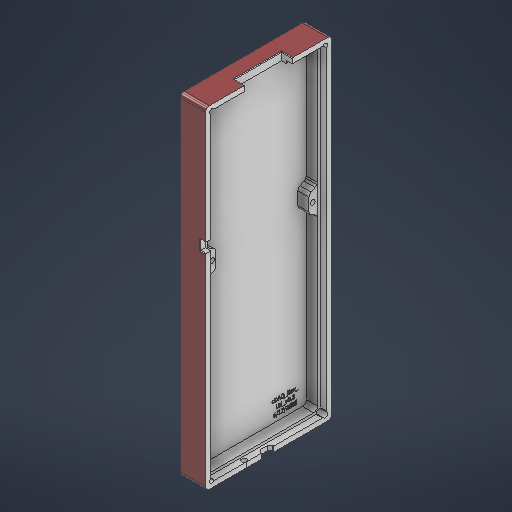
# Autodesk Inventor part: cDAQ_Box_Lid_v0.2
Saved by Autodesk Inventor 2027 (Build 310192000, 192)
## iProperties
Created: 2026-05-08
Part Number: cDAQ_Box_Lid_v0.2
Material: Generic
Document SubType Name: Modeling
Designer: giese
Density: 1 g/cm^3
Appearance: Default
Author: giese
Autodesk Inventor part; units mm, degrees
(part 1 of 2)
ref_plane "YZ Plane" through (0, 0, 0) normal (1, 0, 0) x (0, 1, 0)
ref_plane "XZ Plane" through (0, 0, 0) normal (0, 1, 0) x (-1, 0, 0)
ref_plane "XY Plane" through (0, 0, 0) normal (0, 0, 1) x (1, 0, 0)
sketch "Sketch1" plane through (0, 0, 0) normal (1, 0, 0) x (0, 1, 0)
  line L0 (50.7569, 48.4212) -> (-216.9591, 48.4212)
  line L1 (-216.9591, 48.4212) -> (-216.9591, -53.1788)
  line L2 (-216.9591, -53.1788) -> (50.7569, -53.1788)
  line L3 (50.7569, -53.1788) -> (50.7569, 48.4212)
  point P0 (0, 0)
  dimension "d0" = 101.6
  dimension "d1" = 267.716
  constraints: 8 end point, 2 parallel, 1 horizontal, 1 perpendicular
  measures "d0" distance of L2.end L0.start
  measures "d1" distance of L0.start L0.end
extrude "Extrusion1" add sketch "Sketch1" along normal blind 20.32
sketch "Sketch2" plane through (20.32, 0, 0) normal (1, 0, 0) x (0, 0, -1)
  line L0 (-42.0712, 44.4069) -> (46.8288, 44.4069)
  line L1 (46.8288, 44.4069) -> (46.8288, -210.6091)
  line L2 (46.8288, -210.6091) -> (-42.0712, -210.6091)
  line L3 (-42.0712, -210.6091) -> (-42.0712, 44.4069)
  line L4 (-48.4212, 50.7569) -> (-48.4212, -216.9591) projected
  line L5 (-48.4212, -216.9591) -> (53.1788, -216.9591) projected
  point P0 (0, 0)
  dimension "d4" = 88.9
  dimension "d5" = 255.016
  dimension "d6" = 6.35
  dimension "d7" = 6.35
  constraints: 8 end point, 2 parallel, 1 horizontal, 1 perpendicular
  measures "d4" distance of L0.start L0.end
  measures "d5" distance of L0.end L1.end
  measures "d6" distance between parallel lines of L4 L3
  measures "d7" distance between parallel lines of L5 L2
extrude "Extrusion2" cut sketch "Sketch2" against normal blind 13.97
sketch "Sketch3" plane through (0, 0, 0) normal (-1, 0, 0) x (0, 0, 1)
  circle A0 centre (-30.3188, 7.3229) radius 2
  line L0 (-53.1788, -216.9591) -> (-53.1788, 50.7569) projected
  line L1 (-53.1788, 50.7569) -> (48.4212, 50.7569) projected
  circle A1 centre (-11.82, 7.3229) radius 2
  circle A2 centre (6.6789, 7.3229) radius 2
  point P0 (0, 0)
  dimension "d10" = 22.86
  dimension "d11" = 43.434
  dimension "d12" = 43.434
  dimension "d13" = 18.4988
  dimension "d14" = 4
  dimension "d15" = 4
  dimension "d16" = 43.434
  dimension "d17" = 18.4988
  dimension "d18" = 36.9976
  dimension "d21" = 4
  constraints: 3 centre point
  measures "d10" distance from line of L0 A0.centre
  measures "d11" distance from line of L1 A0.centre
  measures "d12" distance from line of L1 A1.centre
  measures "d13" distance of A0.centre A1.centre
  measures "d14" diameter of A1
  measures "d15" diameter of A2
  measures "d16" distance from line of L1 A2.centre
  measures "d17" distance of A1.centre A2.centre
  measures "d18" distance of A0.centre A2.centre
  measures "d21" diameter of A0
extrude "Extrusion3" [suppressed]
sketch "Sketch6" plane through (0, 50.7569, 48.4212) normal (0, 1, 0) x (1, 0, 0)
  line L0 (20.32, 6.35) -> (20.32, 95.25) projected
  line L1 (11.684, 31.75) -> (20.32, 31.75)
  line L2 (20.32, 31.75) -> (20.32, 69.85)
  line L3 (20.32, 69.85) -> (11.684, 69.85)
  line L4 (11.684, 69.85) -> (11.684, 31.75)
  line L5 (0, 101.6) -> (20.32, 101.6) projected
  point P0 (0, 48.4212)
  point P1 (16.002, 69.85)
  point P2 (16.002, 31.75)
  dimension "d30" = 8.636
  dimension "d31" = 38.1
  dimension "d32" = 31.75
  constraints: 8 end point, 2 midpoint, 2 parallel, 1 horizontal, 1 perpendicular, 1 point on line
  measures "d30" distance between parallel lines of L0 L4
  measures "d31" distance of point (16.002, 69.85) point (16.002, 31.75)
  measures "d32" distance between parallel lines of L5 L3
extrude "Extrusion5" cut sketch "Sketch6" against normal blind 6.35
fillet "Fillet1" radius 3.175 4 edges at (10.16, 50.7569, -53.1788) (10.16, 50.7569, 48.4212) (10.16, -216.9591, 48.4212) (10.16, -216.9591, -53.1788)
sketch "Sketch7" plane through (20.32, 0, 0) normal (1, 0, 0) x (0, 0, -1)
  line L0 (-42.0712, -210.6091) -> (-42.0712, 44.4069) projected
  line L1 (-42.0712, 44.4069) -> (-42.3252, 44.4069)
  line L2 (-42.3252, 46.5659) -> (-44.2302, 46.5659)
  line L3 (-44.2302, 46.5659) -> (-44.2302, 51.0109)
  line L4 (-42.0712, -190.1621) -> (-42.0712, -210.6091)
  line L5 (46.8288, -210.6091) -> (-42.0712, -210.6091) projected
  line L6 (-40.4202, -212.7681) -> (-44.2302, -212.7681)
  line L7 (-44.2302, -212.7681) -> (-44.2302, -190.1621)
  line L8 (46.8288, 44.4069) -> (46.8288, -210.6091) projected
  line L9 (46.8288, -192.7021) -> (46.8288, -210.6091)
  line L10 (46.8288, -210.6091) -> (43.9078, -210.6091)
  line L11 (46.8288, -210.6091) -> (46.8288, -192.7021)
  line L12 (48.9878, -192.7021) -> (48.9878, -212.7681)
  line L13 (48.9878, -212.7681) -> (43.9078, -212.7681)
  line L14 (-42.0712, 44.4069) -> (46.8288, 44.4069) projected
  line L15 (42.0028, 44.4069) -> (46.8288, 44.4069)
  line L16 (48.9878, 48.4709) -> (48.9878, 46.5659)
  line L17 (48.9878, 46.5659) -> (42.0028, 46.5659)
  line L18 (-42.3252, 46.5659) -> (42.0028, 46.5659)
  line L19 (42.0028, 44.4069) -> (-42.3252, 44.4069)
  line L20 (48.9878, 48.4709) -> (48.9878, -192.7021)
  line L21 (44.2888, -195.2421) -> (44.2888, 44.4069)
  line L22 (43.9078, -210.6091) -> (-40.4202, -210.6091)
  line L23 (-40.4202, -212.7681) -> (43.9078, -212.7681)
  line L24 (-44.2302, -190.1621) -> (-44.2302, 51.0109)
  line L25 (-42.0712, 44.4069) -> (-42.0712, -190.1621)
  point P0 (0, 0)
  point P1 (-42.0712, 51.0109)
  point P2 (-44.2302, 48.9789)
  point P3 (46.8288, 48.4709)
  point P4 (48.9878, 46.5659)
  point P5 (-44.2302, 46.5659)
  dimension "d34" = 2.159
  dimension "d35" = 2.159
  dimension "d38" = 2.159
  dimension "d39" = 2.159
  dimension "d42" = 2.159
  dimension "d43" = 2.159
  dimension "d46" = 2.159
  dimension "d47" = 2.159
  constraints: 44 end point, 9 point on line, 4 parallel, 4 perpendicular, 2 collinear, 2 horizontal, 2 vertical
  measures "d34" distance between parallel lines of L2 L1
  measures "d35" distance between parallel lines of L0 L3
  measures "d38" distance between parallel lines of L7 L0
  measures "d39" distance between parallel lines of L5 L6
  measures "d42" distance between parallel lines of L5 L13
  measures "d43" distance between parallel lines of L8 L12
  measures "d46" distance between parallel lines of L14 L17
  measures "d47" distance between parallel lines of L8 L16
extrude "Extrusion6" cut sketch "Sketch7" against normal blind 5 contours L0 L14 L8 L5 | L18 L17 L20 L12 L13 L23 L6 L7 L24 L2
fillet "Fillet2" radius 3.175 6 edges at (10.835, 44.4069, 42.0712) (10.835, 44.4069, -46.8288) (10.835, -210.6091, 42.0712) (17.82, -212.7681, 44.2302) (10.835, -210.6091, -46.8288) (17.82, -212.7681, -48.9878)
sketch "Sketch11" plane through (15.32, 0, 0) normal (1, 0, 0) x (0, 0, -1)
  circle A0 centre (48.0988, 45.6769) radius 1.9939
  line L0 (50.0038, 50.7569) -> (21.4288, 50.7569) projected
  line L1 (53.1788, -213.7841) -> (53.1788, 47.5819) projected
  arc A1 (46.9238, 45.7719) -> (43.7488, 48.9469) centre (43.7488, 45.7719) ccw projected
  circle A2 centre (-43.3412, 45.6769) radius 1.9939
  line L2 (-48.4212, 47.5819) -> (-48.4212, -213.7841) projected
  line L3 (-16.6712, 50.7569) -> (-45.2462, 50.7569) projected
  circle A3 centre (48.0988, -211.8791) radius 1.9939
  line L4 (-45.2462, -216.9591) -> (50.0038, -216.9591) projected
  circle A4 centre (-43.3412, -211.8791) radius 1.9939
  circle A5 centre (43.0188, -63.5431) radius 1.9939
  circle A6 centre (-38.2612, -63.5431) radius 1.9939
  point P0 (0, 0)
  point P1 (45.9939, 48.017)
  point P2 (48.5528, -43.2993)
  point P3 (45.3778, -46.4743)
  point P4 (-30.4007, -42.8803)
  point P5 (-33.5757, -46.0553)
  dimension "d58" = 3.9878
  dimension "d59" = 5.08
  dimension "d60" = 5.08
  dimension "d61" = 3.9878
  dimension "d62" = 3.9878
  dimension "d63" = 5.08
  dimension "d64" = 5.08
  dimension "d65" = 3.9878
  dimension "d66" = 5.08
  dimension "d67" = 5.08
  dimension "d76" = 5.08
  dimension "d77" = 5.08
  dimension "d114" = 3.9878
  dimension "d115" = 114.3
  dimension "d116" = 10.16
  dimension "d117" = 3.9878
  dimension "d118" = 114.3
  dimension "d119" = 10.16
  constraints: 6 centre point, 1 point on circle
  measures "d58" diameter of A0
  measures "d59" distance from line of L2 A2.centre
  measures "d60" distance from line of L3 A2.centre
  measures "d61" diameter of A2
  measures "d62" diameter of A3
  measures "d63" distance from line of L1 A3.centre
  measures "d64" distance from line of L4 A3.centre
  measures "d65" diameter of A4
  measures "d66" distance from line of L2 A4.centre
  measures "d67" distance from line of L4 A4.centre
  measures "d76" distance from line of L1 A0.centre
  measures "d77" distance from line of L0 A0.centre
  measures "d114" diameter of A5
  measures "d115" distance from line of A5.centre L0
  measures "d116" distance from line of L1 A5.centre
  measures "d117" diameter of A6
  measures "d118" distance from line of A6.centre L3
  measures "d119" distance from line of L2 A6.centre
extrude "Extrusion8" cut sketch "Sketch11" along normal blind 5.08 and the other way blind 17.78
sketch "Sketch13" plane through (6.35, 0, 0) normal (1, 0, 0) x (0, 0, -1)
  line L0 (17.2683, -193.8209) -> (42.3242, -193.8209) construction
  line L1 (42.3242, -193.8209) -> (42.3242, -202.6852) construction
  line L2 (42.3242, -202.6852) -> (17.2683, -202.6852) construction
  line L3 (17.2683, -202.6852) -> (17.2683, -193.8209) construction
  spline S0 degree 2 poles (20.1261, -196.985) (19.889, -196.985) (19.4963, -196.8393) (19.3555, -196.6911) knots 0 0 0 1 2 2 2
  spline S1 degree 2 poles (19.3555, -196.6911) (19.2147, -196.5454) (19.0591, -196.0958) (19.0591, -195.7945) knots 0 0 0 1 2 2 2
  spline S2 degree 2 poles (19.0591, -195.7945) (19.0591, -195.4931) (19.2196, -195.0535) (19.3555, -194.9053) knots 0 0 0 1 2 2 2
  spline S3 degree 2 poles (19.3555, -194.9053) (19.4913, -194.7546) (19.8939, -194.5941) (20.1261, -194.5941) knots 0 0 0 1 2 2 2
  spline S4 degree 2 poles (20.1261, -194.5941) (20.3138, -194.5941) (20.6646, -194.7003) (20.8004, -194.7694) knots 0 0 0 1 2 2 2
  line L4 (20.8004, -194.7694) -> (20.8004, -195.2017)
  line L5 (20.8004, -195.2017) -> (20.7782, -195.2017)
  spline S5 degree 2 poles (20.7782, -195.2017) (20.7362, -195.1671) (20.6078, -195.0782) (20.5164, -195.0312) knots 0 0 0 1 2 2 2
  spline S6 degree 2 poles (20.5164, -195.0312) (20.4349, -194.9917) (20.2175, -194.93) (20.1187, -194.93) knots 0 0 0 1 2 2 2
  spline S7 degree 2 poles (20.1187, -194.93) (19.8198, -194.93) (19.4568, -195.382) (19.4568, -195.7945) knots 0 0 0 1 2 2 2
  spline S8 degree 2 poles (19.4568, -195.7945) (19.4568, -196.1971) (19.8075, -196.6491) (20.1187, -196.6491) knots 0 0 0 1 2 2 2
  spline S9 degree 2 poles (20.1187, -196.6491) (20.3064, -196.6491) (20.6473, -196.4935) (20.7782, -196.3725) knots 0 0 0 1 2 2 2
  line L6 (20.7782, -196.3725) -> (20.8004, -196.3725)
  line L7 (20.8004, -196.3725) -> (20.8004, -196.8047)
  spline S10 degree 2 poles (20.8004, -196.8047) (20.7436, -196.8319) (20.5707, -196.9085) (20.5016, -196.9257) knots 0 0 0 1 2 2 2
  spline S11 degree 2 poles (20.5016, -196.9257) (20.4028, -196.9554) (20.2472, -196.985) (20.1261, -196.985) knots 0 0 0 1 2 2 2
  spline S12 degree 2 poles (23.5842, -195.4116) (23.5842, -195.8291) (23.2458, -196.5009) (22.9617, -196.6886) knots 0 0 0 1 2 2 2
  spline S13 degree 2 poles (22.9617, -196.6886) (22.7295, -196.8344) (22.2528, -196.9332) (21.8823, -196.9332) knots 0 0 0 1 2 2 2
  line L8 (21.8823, -196.9332) -> (21.1808, -196.9332)
  line L9 (21.1808, -196.9332) -> (21.1808, -193.8852)
  line L10 (21.1808, -193.8852) -> (21.8749, -193.8852)
  spline S14 degree 2 poles (21.8749, -193.8852) (22.3047, -193.8852) (22.7937, -194.0136) (22.9666, -194.1272) knots 0 0 0 1 2 2 2
  spline S15 degree 2 poles (22.9666, -194.1272) (23.2606, -194.3223) (23.5842, -194.967) (23.5842, -195.4116) knots 0 0 0 1 2 2 2
  spline S16 degree 2 poles (23.1618, -195.4067) (23.1618, -195.0559) (22.9296, -194.5595) (22.6999, -194.4187) knots 0 0 0 1 2 2 2
  spline S17 degree 2 poles (22.6999, -194.4187) (22.5369, -194.3223) (22.1688, -194.2359) (21.8947, -194.2359) knots 0 0 0 1 2 2 2
  line L11 (21.8947, -194.2359) -> (21.5859, -194.2359)
  line L12 (21.5859, -194.2359) -> (21.5859, -196.5824)
  line L13 (21.5859, -196.5824) -> (21.8947, -196.5824)
  spline S18 degree 2 poles (21.8947, -196.5824) (22.1639, -196.5824) (22.5714, -196.496) (22.7369, -196.3799) knots 0 0 0 1 2 2 2
  spline S19 degree 2 poles (22.7369, -196.3799) (22.9494, -196.2366) (23.1618, -195.7624) (23.1618, -195.4067) knots 0 0 0 1 2 2 2
  line L14 (23.6953, -196.9332) -> (24.7228, -193.8852)
  line L15 (24.7228, -193.8852) -> (25.2218, -193.8852)
  line L16 (25.2218, -193.8852) -> (26.2493, -196.9332)
  line L17 (26.2493, -196.9332) -> (25.822, -196.9332)
  line L18 (25.822, -196.9332) -> (25.5453, -196.081)
  line L19 (25.5453, -196.081) -> (24.382, -196.081)
  line L20 (24.382, -196.081) -> (24.1053, -196.9332)
  line L21 (24.1053, -196.9332) -> (23.6953, -196.9332)
  line L22 (25.4342, -195.7352) -> (24.9624, -194.3001)
  line L23 (24.9624, -194.3001) -> (24.4931, -195.7352)
  line L24 (24.4931, -195.7352) -> (25.4342, -195.7352)
  spline S20 degree 2 poles (29.0701, -197.6791) (28.9589, -197.7063) (28.7168, -197.7359) (28.5958, -197.7359) knots 0 0 0 1 2 2 2
  spline S21 degree 2 poles (28.5958, -197.7359) (28.2525, -197.7359) (27.8252, -197.3531) (27.8054, -196.9974) knots 0 0 0 1 2 2 2
  spline S22 degree 2 poles (27.8054, -196.9974) (27.7782, -196.9974) (27.7313, -196.9974) (27.7115, -196.9974) knots 0 0 0 1 2 2 2
  spline S23 degree 2 poles (27.7115, -196.9974) (27.4028, -196.9974) (26.9063, -196.7874) (26.7285, -196.5824) knots 0 0 0 1 2 2 2
  spline S24 degree 2 poles (26.7285, -196.5824) (26.5531, -196.3799) (26.3654, -195.7871) (26.3654, -195.4116) knots 0 0 0 1 2 2 2
  spline S25 degree 2 poles (26.3654, -195.4116) (26.3654, -195.0263) (26.5556, -194.4434) (26.731, -194.2359) knots 0 0 0 1 2 2 2
  spline S26 degree 2 poles (26.731, -194.2359) (26.9088, -194.0309) (27.4053, -193.8209) (27.7115, -193.8209) knots 0 0 0 1 2 2 2
  spline S27 degree 2 poles (27.7115, -193.8209) (28.0228, -193.8209) (28.5217, -194.0383) (28.6946, -194.2359) knots 0 0 0 1 2 2 2
  spline S28 degree 2 poles (28.6946, -194.2359) (28.8675, -194.436) (29.0602, -195.0312) (29.0602, -195.4116) knots 0 0 0 1 2 2 2
  spline S29 degree 2 poles (29.0602, -195.4116) (29.0602, -196.0044) (28.5983, -196.7751) (28.1957, -196.9109) knots 0 0 0 1 2 2 2
  spline S30 degree 2 poles (28.1957, -196.9109) (28.2056, -197.0245) (28.2648, -197.2073) (28.3118, -197.2592) knots 0 0 0 1 2 2 2
  spline S31 degree 2 poles (28.3118, -197.2592) (28.3686, -197.3234) (28.5242, -197.3827) (28.6625, -197.3827) knots 0 0 0 1 2 2 2
  spline S32 degree 2 poles (28.6625, -197.3827) (28.744, -197.3827) (28.9663, -197.3308) (29.0157, -197.3111) knots 0 0 0 1 2 2 2
  line L25 (29.0157, -197.3111) -> (29.0701, -197.3111)
  line L26 (29.0701, -197.3111) -> (29.0701, -197.6791)
  spline S33 degree 2 poles (28.6378, -195.4116) (28.6378, -195.1078) (28.5069, -194.641) (28.3883, -194.4878) knots 0 0 0 1 2 2 2
  spline S34 degree 2 poles (28.3883, -194.4878) (28.2673, -194.3298) (27.9264, -194.1717) (27.714, -194.1717) knots 0 0 0 1 2 2 2
  spline S35 degree 2 poles (27.714, -194.1717) (27.4942, -194.1717) (27.1632, -194.3248) (27.0372, -194.4878) knots 0 0 0 1 2 2 2
  spline S36 degree 2 poles (27.0372, -194.4878) (26.9162, -194.6435) (26.7878, -195.1152) (26.7878, -195.4116) knots 0 0 0 1 2 2 2
  spline S37 degree 2 poles (26.7878, -195.4116) (26.7878, -196.0118) (27.2916, -196.6516) (27.714, -196.6516) knots 0 0 0 1 2 2 2
  spline S38 degree 2 poles (27.714, -196.6516) (28.1364, -196.6516) (28.6378, -196.0118) (28.6378, -195.4116) knots 0 0 0 1 2 2 2
  line L27 (31.5154, -197.5457) -> (29.1639, -197.5457)
  line L28 (29.1639, -197.5457) -> (29.1639, -197.2814)
  line L29 (29.1639, -197.2814) -> (31.5154, -197.2814)
  line L30 (31.5154, -197.2814) -> (31.5154, -197.5457)
  spline S39 degree 2 poles (33.8594, -195.997) (33.8594, -196.2243) (33.6865, -196.5725) (33.5433, -196.6862) knots 0 0 0 1 2 2 2
  spline S40 degree 2 poles (33.5433, -196.6862) (33.3704, -196.8195) (32.9776, -196.9332) (32.6664, -196.9332) knots 0 0 0 1 2 2 2
  line L31 (32.6664, -196.9332) -> (31.792, -196.9332)
  line L32 (31.792, -196.9332) -> (31.792, -193.8852)
  line L33 (31.792, -193.8852) -> (32.5997, -193.8852)
  spline S41 degree 2 poles (32.5997, -193.8852) (32.9258, -193.8852) (33.2518, -193.9271) (33.4, -194.0087) knots 0 0 0 1 2 2 2
  spline S42 degree 2 poles (33.4, -194.0087) (33.5655, -194.0951) (33.7162, -194.3792) (33.7162, -194.5718) knots 0 0 0 1 2 2 2
  spline S43 degree 2 poles (33.7162, -194.5718) (33.7162, -194.7867) (33.4889, -195.1276) (33.2888, -195.2239) knots 0 0 0 1 2 2 2
  line L34 (33.2888, -195.2239) -> (33.2888, -195.2387)
  spline S44 degree 2 poles (33.2888, -195.2387) (33.5605, -195.3128) (33.8594, -195.7056) (33.8594, -195.997) knots 0 0 0 1 2 2 2
  spline S45 degree 2 poles (33.437, -196.0143) (33.437, -195.8414) (33.3382, -195.6191) (33.19, -195.5401) knots 0 0 0 1 2 2 2
  spline S46 degree 2 poles (33.19, -195.5401) (33.0937, -195.4907) (32.8665, -195.461) (32.6565, -195.461) knots 0 0 0 1 2 2 2
  line L35 (32.6565, -195.461) -> (32.1971, -195.461)
  line L36 (32.1971, -195.461) -> (32.1971, -196.5874)
  line L37 (32.1971, -196.5874) -> (32.5256, -196.5874)
  spline S47 degree 2 poles (32.5256, -196.5874) (32.7924, -196.5874) (33.0987, -196.538) (33.2172, -196.4589) knots 0 0 0 1 2 2 2
  spline S48 degree 2 poles (33.2172, -196.4589) (33.3308, -196.3774) (33.437, -196.1749) (33.437, -196.0143) knots 0 0 0 1 2 2 2
  spline S49 degree 2 poles (33.2938, -194.6286) (33.2938, -194.5199) (33.2197, -194.3569) (33.1382, -194.31) knots 0 0 0 1 2 2 2
  spline S50 degree 2 poles (33.1382, -194.31) (33.0394, -194.2557) (32.7998, -194.231) (32.5849, -194.231) knots 0 0 0 1 2 2 2
  line L38 (32.5849, -194.231) -> (32.1971, -194.231)
  line L39 (32.1971, -194.231) -> (32.1971, -195.1226)
  line L40 (32.1971, -195.1226) -> (32.6565, -195.1226)
  spline S51 degree 2 poles (32.6565, -195.1226) (32.8467, -195.1226) (33.027, -195.0831) (33.1234, -195.0214) knots 0 0 0 1 2 2 2
  spline S52 degree 2 poles (33.1234, -195.0214) (33.2172, -194.9621) (33.2938, -194.7719) (33.2938, -194.6286) knots 0 0 0 1 2 2 2
  spline S53 degree 2 poles (36.1121, -195.7895) (36.1121, -196.3675) (35.5563, -196.9974) (35.092, -196.9974) knots 0 0 0 1 2 2 2
  spline S54 degree 2 poles (35.092, -196.9974) (34.6152, -196.9974) (34.0694, -196.3478) (34.0694, -195.7895) knots 0 0 0 1 2 2 2
  spline S55 degree 2 poles (34.0694, -195.7895) (34.0694, -195.2165) (34.6325, -194.5817) (35.092, -194.5817) knots 0 0 0 1 2 2 2
  spline S56 degree 2 poles (35.092, -194.5817) (35.5563, -194.5817) (36.1121, -195.214) (36.1121, -195.7895) knots 0 0 0 1 2 2 2
  spline S57 degree 2 poles (35.7144, -195.7895) (35.7144, -195.3449) (35.3908, -194.9127) (35.092, -194.9127) knots 0 0 0 1 2 2 2
  spline S58 degree 2 poles (35.092, -194.9127) (34.7931, -194.9127) (34.467, -195.3449) (34.467, -195.7895) knots 0 0 0 1 2 2 2
  spline S59 degree 2 poles (34.467, -195.7895) (34.467, -196.2218) (34.7931, -196.6664) (35.092, -196.6664) knots 0 0 0 1 2 2 2
  spline S60 degree 2 poles (35.092, -196.6664) (35.3884, -196.6664) (35.7144, -196.2292) (35.7144, -195.7895) knots 0 0 0 1 2 2 2
  line L41 (38.2832, -196.9332) -> (37.8114, -196.9332)
  line L42 (37.8114, -196.9332) -> (37.2557, -196.0736)
  line L43 (37.2557, -196.0736) -> (36.6851, -196.9332)
  line L44 (36.6851, -196.9332) -> (36.2479, -196.9332)
  line L45 (36.2479, -196.9332) -> (37.0408, -195.7994)
  line L46 (37.0408, -195.7994) -> (36.2553, -194.6459)
  line L47 (36.2553, -194.6459) -> (36.7271, -194.6459)
  line L48 (36.7271, -194.6459) -> (37.2804, -195.4981)
  line L49 (37.2804, -195.4981) -> (37.846, -194.6459)
  line L50 (37.846, -194.6459) -> (38.2832, -194.6459)
  line L51 (38.2832, -194.6459) -> (37.4953, -195.7747)
  line L52 (37.4953, -195.7747) -> (38.2832, -196.9332)
  line L53 (40.6223, -197.5457) -> (38.2709, -197.5457)
  line L54 (38.2709, -197.5457) -> (38.2709, -197.2814)
  line L55 (38.2709, -197.2814) -> (40.6223, -197.2814)
  line L56 (40.6223, -197.2814) -> (40.6223, -197.5457)
  line L57 (24.0819, -201.9516) -> (22.3158, -201.9516)
  line L58 (22.3158, -201.9516) -> (22.3158, -198.9036)
  line L59 (22.3158, -198.9036) -> (22.7209, -198.9036)
  line L60 (22.7209, -198.9036) -> (22.7209, -201.591)
  line L61 (22.7209, -201.591) -> (24.0819, -201.591)
  line L62 (24.0819, -201.591) -> (24.0819, -201.9516)
  line L63 (24.7636, -201.9516) -> (24.3783, -201.9516)
  line L64 (24.3783, -201.9516) -> (24.3783, -199.6644)
  line L65 (24.3783, -199.6644) -> (24.7636, -199.6644)
  line L66 (24.7636, -199.6644) -> (24.7636, -201.9516)
  line L67 (24.7908, -199.284) -> (24.3536, -199.284)
  line L68 (24.3536, -199.284) -> (24.3536, -198.8838)
  line L69 (24.3536, -198.8838) -> (24.7908, -198.8838)
  line L70 (24.7908, -198.8838) -> (24.7908, -199.284)
  line L71 (27.0879, -201.9516) -> (26.7025, -201.9516)
  line L72 (26.7025, -201.9516) -> (26.7025, -201.7194)
  spline S61 degree 2 poles (26.7025, -201.7194) (26.6136, -201.7935) (26.4827, -201.8923) (26.3938, -201.9343) knots 0 0 0 1 2 2 2
  spline S62 degree 2 poles (26.3938, -201.9343) (26.3123, -201.9738) (26.1369, -202.0158) (26.0208, -202.0158) knots 0 0 0 1 2 2 2
  spline S63 degree 2 poles (26.0208, -202.0158) (25.8331, -202.0158) (25.5169, -201.8602) (25.4058, -201.7095) knots 0 0 0 1 2 2 2
  spline S64 degree 2 poles (25.4058, -201.7095) (25.2946, -201.5589) (25.1711, -201.1143) (25.1711, -200.8253) knots 0 0 0 1 2 2 2
  spline S65 degree 2 poles (25.1711, -200.8253) (25.1711, -200.5239) (25.3267, -200.0843) (25.4626, -199.9188) knots 0 0 0 1 2 2 2
  spline S66 degree 2 poles (25.4626, -199.9188) (25.5886, -199.7706) (25.9418, -199.6002) (26.1369, -199.6002) knots 0 0 0 1 2 2 2
  spline S67 degree 2 poles (26.1369, -199.6002) (26.3073, -199.6002) (26.5618, -199.6767) (26.7025, -199.7558) knots 0 0 0 1 2 2 2
  line L73 (26.7025, -199.7558) -> (26.7025, -198.7678)
  line L74 (26.7025, -198.7678) -> (27.0879, -198.7678)
  line L75 (27.0879, -198.7678) -> (27.0879, -201.9516)
  line L76 (26.7025, -201.3959) -> (26.7025, -200.0744)
  spline S68 degree 2 poles (26.7025, -200.0744) (26.5593, -200.0052) (26.332, -199.9534) (26.2011, -199.9534) knots 0 0 0 1 2 2 2
  spline S69 degree 2 poles (26.2011, -199.9534) (25.9047, -199.9534) (25.5688, -200.398) (25.5688, -200.8179) knots 0 0 0 1 2 2 2
  spline S70 degree 2 poles (25.5688, -200.8179) (25.5688, -201.223) (25.8257, -201.6503) (26.1097, -201.6503) knots 0 0 0 1 2 2 2
  spline S71 degree 2 poles (26.1097, -201.6503) (26.2604, -201.6503) (26.5667, -201.5119) (26.7025, -201.3959) knots 0 0 0 1 2 2 2
  line L77 (29.6863, -202.5642) -> (27.3349, -202.5642)
  line L78 (27.3349, -202.5642) -> (27.3349, -202.2999)
  line L79 (27.3349, -202.2999) -> (29.6863, -202.2999)
  line L80 (29.6863, -202.2999) -> (29.6863, -202.5642)
  line L81 (31.729, -199.6644) -> (30.867, -201.9516)
  line L82 (30.867, -201.9516) -> (30.5212, -201.9516)
  line L83 (30.5212, -201.9516) -> (29.6666, -199.6644)
  line L84 (29.6666, -199.6644) -> (30.084, -199.6644)
  line L85 (30.084, -199.6644) -> (30.7089, -201.4255)
  line L86 (30.7089, -201.4255) -> (31.3289, -199.6644)
  line L87 (31.3289, -199.6644) -> (31.729, -199.6644)
  spline S72 degree 2 poles (33.8607, -200.4276) (33.8607, -201.2477) (33.3839, -202.0158) (32.8875, -202.0158) knots 0 0 0 1 2 2 2
  spline S73 degree 2 poles (32.8875, -202.0158) (32.3836, -202.0158) (31.9118, -201.2328) (31.9118, -200.4301) knots 0 0 0 1 2 2 2
  spline S74 degree 2 poles (31.9118, -200.4301) (31.9118, -199.6051) (32.3885, -198.8419) (32.8875, -198.8419) knots 0 0 0 1 2 2 2
  spline S75 degree 2 poles (32.8875, -198.8419) (33.3889, -198.8419) (33.8607, -199.6323) (33.8607, -200.4276) knots 0 0 0 1 2 2 2
  spline S76 degree 2 poles (33.337, -201.3563) (33.3963, -201.2057) (33.4457, -200.7413) (33.4457, -200.4276) knots 0 0 0 1 2 2 2
  spline S77 degree 2 poles (33.4457, -200.4276) (33.4457, -200.1139) (33.3963, -199.652) (33.3345, -199.4964) knots 0 0 0 1 2 2 2
  spline S78 degree 2 poles (33.3345, -199.4964) (33.2728, -199.3408) (33.0579, -199.1802) (32.8875, -199.1802) knots 0 0 0 1 2 2 2
  spline S79 degree 2 poles (32.8875, -199.1802) (32.717, -199.1802) (32.4972, -199.3408) (32.433, -199.5014) knots 0 0 0 1 2 2 2
  spline S80 degree 2 poles (32.433, -199.5014) (32.3712, -199.657) (32.3268, -200.1312) (32.3268, -200.4301) knots 0 0 0 1 2 2 2
  spline S81 degree 2 poles (32.3268, -200.4301) (32.3268, -200.7512) (32.3663, -201.181) (32.4305, -201.3489) knots 0 0 0 1 2 2 2
  spline S82 degree 2 poles (32.4305, -201.3489) (32.4898, -201.507) (32.7096, -201.6774) (32.8875, -201.6774) knots 0 0 0 1 2 2 2
  spline S83 degree 2 poles (32.8875, -201.6774) (33.0554, -201.6774) (33.2753, -201.5169) (33.337, -201.3563) knots 0 0 0 1 2 2 2
  line L88 (34.9055, -201.9516) -> (34.4164, -201.9516)
  line L89 (34.4164, -201.9516) -> (34.4164, -201.3687)
  line L90 (34.4164, -201.3687) -> (34.9055, -201.3687)
  line L91 (34.9055, -201.3687) -> (34.9055, -201.9516)
  line L92 (37.4002, -201.9516) -> (35.5205, -201.9516)
  line L93 (35.5205, -201.9516) -> (35.5205, -201.5194)
  spline S84 degree 2 poles (35.5205, -201.5194) (35.723, -201.3292) (36.0837, -200.976) (36.2566, -200.7858) knots 0 0 0 1 2 2 2
  spline S85 degree 2 poles (36.2566, -200.7858) (36.6048, -200.4029) (36.8593, -199.9435) (36.8593, -199.699) knots 0 0 0 1 2 2 2
  spline S86 degree 2 poles (36.8593, -199.699) (36.8593, -199.5705) (36.7802, -199.3779) (36.7086, -199.3161) knots 0 0 0 1 2 2 2
  spline S87 degree 2 poles (36.7086, -199.3161) (36.637, -199.2543) (36.4492, -199.1926) (36.3356, -199.1926) knots 0 0 0 1 2 2 2
  spline S88 degree 2 poles (36.3356, -199.1926) (36.2269, -199.1926) (36.0046, -199.2469) (35.9034, -199.2889) knots 0 0 0 1 2 2 2
  spline S89 degree 2 poles (35.9034, -199.2889) (35.8169, -199.3235) (35.6564, -199.4223) (35.607, -199.4569) knots 0 0 0 1 2 2 2
  line L94 (35.607, -199.4569) -> (35.5847, -199.4569)
  line L95 (35.5847, -199.4569) -> (35.5847, -199.0222)
  spline S90 degree 2 poles (35.5847, -199.0222) (35.7107, -198.9604) (36.1627, -198.8394) (36.3653, -198.8394) knots 0 0 0 1 2 2 2
  spline S91 degree 2 poles (36.3653, -198.8394) (36.7926, -198.8394) (37.2742, -199.2914) (37.2742, -199.6767) knots 0 0 0 1 2 2 2
  spline S92 degree 2 poles (37.2742, -199.6767) (37.2742, -199.857) (37.1902, -200.1584) (37.1161, -200.2868) knots 0 0 0 1 2 2 2
  spline S93 degree 2 poles (37.1161, -200.2868) (37.042, -200.4202) (36.8271, -200.682) (36.7086, -200.808) knots 0 0 0 1 2 2 2
  spline S94 degree 2 poles (36.7086, -200.808) (36.5159, -201.0179) (36.0441, -201.4675) (35.9034, -201.5984) knots 0 0 0 1 2 2 2
  line L96 (35.9034, -201.5984) -> (37.4002, -201.5984)
  line L97 (37.4002, -201.5984) -> (37.4002, -201.9516)
  spline S95 degree 2 poles (22.3368, -205.9821) (22.3368, -206.2167) (22.1812, -206.6144) (22.0503, -206.7478) knots 0 0 0 1 2 2 2
  spline S96 degree 2 poles (22.0503, -206.7478) (21.9144, -206.8885) (21.5736, -207.0343) (21.3685, -207.0343) knots 0 0 0 1 2 2 2
  spline S97 degree 2 poles (21.3685, -207.0343) (21.1635, -207.0343) (20.8251, -206.896) (20.6967, -206.7576) knots 0 0 0 1 2 2 2
  spline S98 degree 2 poles (20.6967, -206.7576) (20.5386, -206.5921) (20.3608, -206.0364) (20.3608, -205.6313) knots 0 0 0 1 2 2 2
  spline S99 degree 2 poles (20.3608, -205.6313) (20.3608, -205.2336) (20.5238, -204.5939) (20.6942, -204.3568) knots 0 0 0 1 2 2 2
  spline S100 degree 2 poles (20.6942, -204.3568) (20.8597, -204.1246) (21.3834, -203.8652) (21.7267, -203.8652) knots 0 0 0 1 2 2 2
  spline S101 degree 2 poles (21.7267, -203.8652) (21.828, -203.8652) (22.0058, -203.885) (22.0725, -203.9072) knots 0 0 0 1 2 2 2
  line L98 (22.0725, -203.9072) -> (22.0725, -204.3)
  line L99 (22.0725, -204.3) -> (22.0552, -204.3)
  spline S102 degree 2 poles (22.0552, -204.3) (21.9984, -204.2703) (21.7909, -204.2185) (21.6724, -204.2185) knots 0 0 0 1 2 2 2
  spline S103 degree 2 poles (21.6724, -204.2185) (21.292, -204.2185) (20.8251, -204.7322) (20.7807, -205.2361) knots 0 0 0 1 2 2 2
  spline S104 degree 2 poles (20.7807, -205.2361) (20.9264, -205.1348) (21.2327, -205.0237) (21.4155, -205.0237) knots 0 0 0 1 2 2 2
  spline S105 degree 2 poles (21.4155, -205.0237) (21.5933, -205.0237) (21.8601, -205.0953) (22.0058, -205.204) knots 0 0 0 1 2 2 2
  spline S106 degree 2 poles (22.0058, -205.204) (22.1738, -205.33) (22.3368, -205.7202) (22.3368, -205.9821) knots 0 0 0 1 2 2 2
  spline S107 degree 2 poles (21.9218, -205.9993) (21.9218, -205.8116) (21.823, -205.5572) (21.7143, -205.4683) knots 0 0 0 1 2 2 2
  spline S108 degree 2 poles (21.7143, -205.4683) (21.6328, -205.4041) (21.4303, -205.3621) (21.3241, -205.3621) knots 0 0 0 1 2 2 2
  spline S109 degree 2 poles (21.3241, -205.3621) (21.1808, -205.3621) (20.9116, -205.4485) (20.7807, -205.53) knots 0 0 0 1 2 2 2
  spline S110 degree 2 poles (20.7807, -205.53) (20.7782, -205.5745) (20.7733, -205.6585) (20.7733, -205.7227) knots 0 0 0 1 2 2 2
  spline S111 degree 2 poles (20.7733, -205.7227) (20.7733, -206.0389) (20.8968, -206.4267) (20.9906, -206.5279) knots 0 0 0 1 2 2 2
  spline S112 degree 2 poles (20.9906, -206.5279) (21.0771, -206.6243) (21.2648, -206.7008) (21.371, -206.7008) knots 0 0 0 1 2 2 2
  spline S113 degree 2 poles (21.371, -206.7008) (21.618, -206.7008) (21.9218, -206.3501) (21.9218, -205.9993) knots 0 0 0 1 2 2 2
  line L100 (23.9645, -203.7862) -> (22.7715, -207.632)
  line L101 (22.7715, -207.632) -> (22.4257, -207.632)
  line L102 (22.4257, -207.632) -> (23.6138, -203.7862)
  line L103 (23.6138, -203.7862) -> (23.9645, -203.7862)
  line L104 (26.027, -206.9701) -> (24.54, -206.9701)
  line L105 (24.54, -206.9701) -> (24.54, -206.6588)
  line L106 (24.54, -206.6588) -> (25.0933, -206.6588)
  line L107 (25.0933, -206.6588) -> (25.0933, -204.6161)
  line L108 (25.0933, -204.6161) -> (24.54, -204.6161)
  line L109 (24.54, -204.6161) -> (24.54, -204.337)
  spline S114 degree 2 poles (24.54, -204.337) (24.8537, -204.337) (25.1501, -204.1592) (25.1699, -203.9122) knots 0 0 0 1 2 2 2
  line L110 (25.1699, -203.9122) -> (25.4861, -203.9122)
  line L111 (25.4861, -203.9122) -> (25.4861, -206.6588)
  line L112 (25.4861, -206.6588) -> (26.027, -206.6588)
  line L113 (26.027, -206.6588) -> (26.027, -206.9701)
  line L114 (28.502, -204.379) -> (27.183, -206.9701)
  line L115 (27.183, -206.9701) -> (26.7482, -206.9701)
  line L116 (26.7482, -206.9701) -> (28.1413, -204.2802)
  line L117 (28.1413, -204.2802) -> (26.5679, -204.2802)
  line L118 (26.5679, -204.2802) -> (26.5679, -203.9221)
  line L119 (26.5679, -203.9221) -> (28.502, -203.9221)
  line L120 (28.502, -203.9221) -> (28.502, -204.379)
  line L121 (30.142, -203.7862) -> (28.949, -207.632)
  line L122 (28.949, -207.632) -> (28.6032, -207.632)
  line L123 (28.6032, -207.632) -> (29.7913, -203.7862)
  line L124 (29.7913, -203.7862) -> (30.142, -203.7862)
  line L125 (32.3576, -206.9701) -> (30.478, -206.9701)
  line L126 (30.478, -206.9701) -> (30.478, -206.5378)
  spline S115 degree 2 poles (30.478, -206.5378) (30.6805, -206.3476) (31.0411, -205.9944) (31.214, -205.8042) knots 0 0 0 1 2 2 2
  spline S116 degree 2 poles (31.214, -205.8042) (31.5623, -205.4214) (31.8167, -204.9619) (31.8167, -204.7174) knots 0 0 0 1 2 2 2
  spline S117 degree 2 poles (31.8167, -204.7174) (31.8167, -204.589) (31.7377, -204.3963) (31.666, -204.3346) knots 0 0 0 1 2 2 2
  spline S118 degree 2 poles (31.666, -204.3346) (31.5944, -204.2728) (31.4067, -204.2111) (31.2931, -204.2111) knots 0 0 0 1 2 2 2
  spline S119 degree 2 poles (31.2931, -204.2111) (31.1844, -204.2111) (30.9621, -204.2654) (30.8608, -204.3074) knots 0 0 0 1 2 2 2
  spline S120 degree 2 poles (30.8608, -204.3074) (30.7744, -204.342) (30.6138, -204.4408) (30.5644, -204.4753) knots 0 0 0 1 2 2 2
  line L127 (30.5644, -204.4753) -> (30.5422, -204.4753)
  line L128 (30.5422, -204.4753) -> (30.5422, -204.0406)
  spline S121 degree 2 poles (30.5422, -204.0406) (30.6682, -203.9789) (31.1202, -203.8578) (31.3227, -203.8578) knots 0 0 0 1 2 2 2
  spline S122 degree 2 poles (31.3227, -203.8578) (31.75, -203.8578) (32.2317, -204.3099) (32.2317, -204.6952) knots 0 0 0 1 2 2 2
  spline S123 degree 2 poles (32.2317, -204.6952) (32.2317, -204.8755) (32.1477, -205.1768) (32.0736, -205.3053) knots 0 0 0 1 2 2 2
  spline S124 degree 2 poles (32.0736, -205.3053) (31.9995, -205.4386) (31.7846, -205.7005) (31.666, -205.8264) knots 0 0 0 1 2 2 2
  spline S125 degree 2 poles (31.666, -205.8264) (31.4734, -206.0364) (31.0016, -206.4859) (30.8608, -206.6168) knots 0 0 0 1 2 2 2
  line L129 (30.8608, -206.6168) -> (32.3576, -206.6168)
  line L130 (32.3576, -206.6168) -> (32.3576, -206.9701)
  spline S126 degree 2 poles (34.6622, -205.4461) (34.6622, -206.2661) (34.1855, -207.0343) (33.689, -207.0343) knots 0 0 0 1 2 2 2
  spline S127 degree 2 poles (33.689, -207.0343) (33.1851, -207.0343) (32.7133, -206.2513) (32.7133, -205.4485) knots 0 0 0 1 2 2 2
  spline S128 degree 2 poles (32.7133, -205.4485) (32.7133, -204.6235) (33.19, -203.8603) (33.689, -203.8603) knots 0 0 0 1 2 2 2
  spline S129 degree 2 poles (33.689, -203.8603) (34.1904, -203.8603) (34.6622, -204.6507) (34.6622, -205.4461) knots 0 0 0 1 2 2 2
  spline S130 degree 2 poles (34.1385, -206.3748) (34.1978, -206.2241) (34.2472, -205.7598) (34.2472, -205.4461) knots 0 0 0 1 2 2 2
  spline S131 degree 2 poles (34.2472, -205.4461) (34.2472, -205.1324) (34.1978, -204.6705) (34.1361, -204.5149) knots 0 0 0 1 2 2 2
  spline S132 degree 2 poles (34.1361, -204.5149) (34.0743, -204.3593) (33.8594, -204.1987) (33.689, -204.1987) knots 0 0 0 1 2 2 2
  spline S133 degree 2 poles (33.689, -204.1987) (33.5186, -204.1987) (33.2987, -204.3593) (33.2345, -204.5198) knots 0 0 0 1 2 2 2
  spline S134 degree 2 poles (33.2345, -204.5198) (33.1728, -204.6754) (33.1283, -205.1497) (33.1283, -205.4485) knots 0 0 0 1 2 2 2
  spline S135 degree 2 poles (33.1283, -205.4485) (33.1283, -205.7696) (33.1678, -206.1994) (33.232, -206.3674) knots 0 0 0 1 2 2 2
  spline S136 degree 2 poles (33.232, -206.3674) (33.2913, -206.5255) (33.5111, -206.6959) (33.689, -206.6959) knots 0 0 0 1 2 2 2
  spline S137 degree 2 poles (33.689, -206.6959) (33.8569, -206.6959) (34.0768, -206.5353) (34.1385, -206.3748) knots 0 0 0 1 2 2 2
  line L131 (36.9321, -206.9701) -> (35.0524, -206.9701)
  line L132 (35.0524, -206.9701) -> (35.0524, -206.5378)
  spline S138 degree 2 poles (35.0524, -206.5378) (35.255, -206.3476) (35.6156, -205.9944) (35.7885, -205.8042) knots 0 0 0 1 2 2 2
  spline S139 degree 2 poles (35.7885, -205.8042) (36.1368, -205.4214) (36.3912, -204.9619) (36.3912, -204.7174) knots 0 0 0 1 2 2 2
  spline S140 degree 2 poles (36.3912, -204.7174) (36.3912, -204.589) (36.3121, -204.3963) (36.2405, -204.3346) knots 0 0 0 1 2 2 2
  spline S141 degree 2 poles (36.2405, -204.3346) (36.1689, -204.2728) (35.9812, -204.2111) (35.8675, -204.2111) knots 0 0 0 1 2 2 2
  spline S142 degree 2 poles (35.8675, -204.2111) (35.7589, -204.2111) (35.5366, -204.2654) (35.4353, -204.3074) knots 0 0 0 1 2 2 2
  spline S143 degree 2 poles (35.4353, -204.3074) (35.3488, -204.342) (35.1883, -204.4408) (35.1389, -204.4753) knots 0 0 0 1 2 2 2
  line L133 (35.1389, -204.4753) -> (35.1167, -204.4753)
  line L134 (35.1167, -204.4753) -> (35.1167, -204.0406)
  spline S144 degree 2 poles (35.1167, -204.0406) (35.2426, -203.9789) (35.6946, -203.8578) (35.8972, -203.8578) knots 0 0 0 1 2 2 2
  spline S145 degree 2 poles (35.8972, -203.8578) (36.3245, -203.8578) (36.8061, -204.3099) (36.8061, -204.6952) knots 0 0 0 1 2 2 2
  spline S146 degree 2 poles (36.8061, -204.6952) (36.8061, -204.8755) (36.7222, -205.1768) (36.6481, -205.3053) knots 0 0 0 1 2 2 2
  spline S147 degree 2 poles (36.6481, -205.3053) (36.574, -205.4386) (36.3591, -205.7005) (36.2405, -205.8264) knots 0 0 0 1 2 2 2
  spline S148 degree 2 poles (36.2405, -205.8264) (36.0479, -206.0364) (35.5761, -206.4859) (35.4353, -206.6168) knots 0 0 0 1 2 2 2
  line L135 (35.4353, -206.6168) -> (36.9321, -206.6168)
  line L136 (36.9321, -206.6168) -> (36.9321, -206.9701)
  spline S149 degree 2 poles (39.2663, -205.9821) (39.2663, -206.2167) (39.1107, -206.6144) (38.9798, -206.7478) knots 0 0 0 1 2 2 2
  spline S150 degree 2 poles (38.9798, -206.7478) (38.8439, -206.8885) (38.503, -207.0343) (38.298, -207.0343) knots 0 0 0 1 2 2 2
  spline S151 degree 2 poles (38.298, -207.0343) (38.093, -207.0343) (37.7546, -206.896) (37.6262, -206.7576) knots 0 0 0 1 2 2 2
  spline S152 degree 2 poles (37.6262, -206.7576) (37.4681, -206.5921) (37.2903, -206.0364) (37.2903, -205.6313) knots 0 0 0 1 2 2 2
  spline S153 degree 2 poles (37.2903, -205.6313) (37.2903, -205.2336) (37.4533, -204.5939) (37.6237, -204.3568) knots 0 0 0 1 2 2 2
  spline S154 degree 2 poles (37.6237, -204.3568) (37.7892, -204.1246) (38.3129, -203.8652) (38.6562, -203.8652) knots 0 0 0 1 2 2 2
  spline S155 degree 2 poles (38.6562, -203.8652) (38.7575, -203.8652) (38.9353, -203.885) (39.002, -203.9072) knots 0 0 0 1 2 2 2
  line L137 (39.002, -203.9072) -> (39.002, -204.3)
  line L138 (39.002, -204.3) -> (38.9847, -204.3)
  spline S156 degree 2 poles (38.9847, -204.3) (38.9279, -204.2703) (38.7204, -204.2185) (38.6018, -204.2185) knots 0 0 0 1 2 2 2
  spline S157 degree 2 poles (38.6018, -204.2185) (38.2215, -204.2185) (37.7546, -204.7322) (37.7102, -205.2361) knots 0 0 0 1 2 2 2
  spline S158 degree 2 poles (37.7102, -205.2361) (37.8559, -205.1348) (38.1622, -205.0237) (38.345, -205.0237) knots 0 0 0 1 2 2 2
  spline S159 degree 2 poles (38.345, -205.0237) (38.5228, -205.0237) (38.7896, -205.0953) (38.9353, -205.204) knots 0 0 0 1 2 2 2
  spline S160 degree 2 poles (38.9353, -205.204) (39.1033, -205.33) (39.2663, -205.7202) (39.2663, -205.9821) knots 0 0 0 1 2 2 2
  spline S161 degree 2 poles (38.8513, -205.9993) (38.8513, -205.8116) (38.7525, -205.5572) (38.6438, -205.4683) knots 0 0 0 1 2 2 2
  spline S162 degree 2 poles (38.6438, -205.4683) (38.5623, -205.4041) (38.3598, -205.3621) (38.2536, -205.3621) knots 0 0 0 1 2 2 2
  spline S163 degree 2 poles (38.2536, -205.3621) (38.1103, -205.3621) (37.8411, -205.4485) (37.7102, -205.53) knots 0 0 0 1 2 2 2
  spline S164 degree 2 poles (37.7102, -205.53) (37.7077, -205.5745) (37.7028, -205.6585) (37.7028, -205.7227) knots 0 0 0 1 2 2 2
  spline S165 degree 2 poles (37.7028, -205.7227) (37.7028, -206.0389) (37.8263, -206.4267) (37.9201, -206.5279) knots 0 0 0 1 2 2 2
  spline S166 degree 2 poles (37.9201, -206.5279) (38.0066, -206.6243) (38.1943, -206.7008) (38.3005, -206.7008) knots 0 0 0 1 2 2 2
  spline S167 degree 2 poles (38.3005, -206.7008) (38.5475, -206.7008) (38.8513, -206.3501) (38.8513, -205.9993) knots 0 0 0 1 2 2 2
  point P0 (0, 0)
  constraints: 2 other
emboss "Emboss1" sketch "Sketch13" operation cut depth 2.54 direction (-1, 0, 0)
sketch "Sketch14" plane through (0, 0, 0) normal (-1, 0, 0) x (0, 0, 1)
  line L0 (-10.4499, -187.9273) -> (8.7669, -187.9273) construction
  line L1 (8.7669, -187.9273) -> (8.7669, -196.7101) construction
  line L2 (8.7669, -196.7101) -> (-10.4499, -196.7101) construction
  line L3 (-10.4499, -196.7101) -> (-10.4499, -187.9273) construction
  line L4 (-23.4175, -195.887) -> (-20.8486, -188.267)
  line L5 (-20.8486, -188.267) -> (-19.6013, -188.267)
  line L6 (-19.6013, -188.267) -> (-17.0325, -195.887)
  line L7 (-17.0325, -195.887) -> (-18.1008, -195.887)
  line L8 (-18.1008, -195.887) -> (-18.7924, -193.7566)
  line L9 (-18.7924, -193.7566) -> (-21.7008, -193.7566)
  line L10 (-21.7008, -193.7566) -> (-22.3924, -195.887)
  line L11 (-22.3924, -195.887) -> (-23.4175, -195.887)
  line L12 (-19.0702, -192.8921) -> (-20.2497, -189.3044)
  line L13 (-20.2497, -189.3044) -> (-21.4229, -192.8921)
  line L14 (-21.4229, -192.8921) -> (-19.0702, -192.8921)
  line L15 (-10.4128, -195.887) -> (-11.7281, -195.887)
  line L16 (-11.7281, -195.887) -> (-14.1364, -192.855)
  line L17 (-14.1364, -192.855) -> (-15.2973, -192.855)
  line L18 (-15.2973, -192.855) -> (-15.2973, -195.887)
  line L19 (-15.2973, -195.887) -> (-16.31, -195.887)
  line L20 (-16.31, -195.887) -> (-16.31, -188.267)
  line L21 (-16.31, -188.267) -> (-14.3463, -188.267)
  spline S0 degree 2 poles (-14.3463, -188.267) (-13.6918, -188.267) (-12.8087, -188.409) (-12.4074, -188.6683) knots 0 0 0 1 2 2 2
  spline S1 degree 2 poles (-12.4074, -188.6683) (-12.006, -188.9277) (-11.5429, -189.7366) (-11.5429, -190.3356) knots 0 0 0 1 2 2 2
  spline S2 degree 2 poles (-11.5429, -190.3356) (-11.5429, -191.1692) (-12.395, -192.2993) (-13.1237, -192.571) knots 0 0 0 1 2 2 2
  line L22 (-13.1237, -192.571) -> (-10.4128, -195.887)
  spline S3 degree 2 poles (-12.5988, -190.4159) (-12.5988, -190.0824) (-12.8334, -189.5699) (-13.0804, -189.4032) knots 0 0 0 1 2 2 2
  spline S4 degree 2 poles (-13.0804, -189.4032) (-13.2966, -189.2612) (-13.8708, -189.1438) (-14.2907, -189.1438) knots 0 0 0 1 2 2 2
  line L23 (-14.2907, -189.1438) -> (-15.2973, -189.1438)
  line L24 (-15.2973, -189.1438) -> (-15.2973, -192.009)
  line L25 (-15.2973, -192.009) -> (-14.4081, -192.009)
  spline S5 degree 2 poles (-14.4081, -192.009) (-13.9696, -192.009) (-13.2719, -191.8547) (-13.031, -191.6138) knots 0 0 0 1 2 2 2
  spline S6 degree 2 poles (-13.031, -191.6138) (-12.8087, -191.4039) (-12.5988, -190.8111) (-12.5988, -190.4159) knots 0 0 0 1 2 2 2
  line L26 (-8.0293, -195.887) -> (-8.0293, -189.1685)
  line L27 (-8.0293, -189.1685) -> (-10.5857, -189.1685)
  line L28 (-10.5857, -189.1685) -> (-10.5857, -188.267)
  line L29 (-10.5857, -188.267) -> (-4.4601, -188.267)
  line L30 (-4.4601, -188.267) -> (-4.4601, -189.1685)
  line L31 (-4.4601, -189.1685) -> (-7.0166, -189.1685)
  line L32 (-7.0166, -189.1685) -> (-7.0166, -195.887)
  line L33 (-7.0166, -195.887) -> (-8.0293, -195.887)
  spline S7 degree 2 poles (-1.564, -196.0228) (-2.3914, -196.0228) (-3.5524, -195.677) (-4.0649, -195.43) knots 0 0 0 1 2 2 2
  line L34 (-4.0649, -195.43) -> (-4.0649, -194.158)
  line L35 (-4.0649, -194.158) -> (-3.9908, -194.158)
  spline S8 degree 2 poles (-3.9908, -194.158) (-3.4906, -194.6273) (-2.2247, -195.146) (-1.6381, -195.146) knots 0 0 0 1 2 2 2
  spline S9 degree 2 poles (-1.6381, -195.146) (-0.7983, -195.146) (0.06, -194.4482) (0.06, -193.8739) knots 0 0 0 1 2 2 2
  spline S10 degree 2 poles (0.06, -193.8739) (0.06, -193.417) (-0.3907, -192.8489) (-0.8786, -192.7068) knots 0 0 0 1 2 2 2
  spline S11 degree 2 poles (-0.8786, -192.7068) (-1.2305, -192.608) (-1.8172, -192.4722) (-2.2556, -192.361) knots 0 0 0 1 2 2 2
  spline S12 degree 2 poles (-2.2556, -192.361) (-2.6508, -192.256) (-3.2745, -191.9411) (-3.5153, -191.6879) knots 0 0 0 1 2 2 2
  spline S13 degree 2 poles (-3.5153, -191.6879) (-3.75, -191.4348) (-4.0093, -190.7555) (-4.0093, -190.3109) knots 0 0 0 1 2 2 2
  spline S14 degree 2 poles (-4.0093, -190.3109) (-4.0093, -189.3847) (-2.5643, -188.1311) (-1.4467, -188.1311) knots 0 0 0 1 2 2 2
  spline S15 degree 2 poles (-1.4467, -188.1311) (-0.8045, -188.1311) (0.3317, -188.3843) (0.8196, -188.6251) knots 0 0 0 1 2 2 2
  line L36 (0.8196, -188.6251) -> (0.8196, -189.8354)
  line L37 (0.8196, -189.8354) -> (0.7455, -189.8354)
  spline S16 degree 2 poles (0.7455, -189.8354) (0.3811, -189.502) (-0.7551, -189.008) (-1.3787, -189.008) knots 0 0 0 1 2 2 2
  spline S17 degree 2 poles (-1.3787, -189.008) (-2.0827, -189.008) (-2.9534, -189.6687) (-2.9534, -190.2059) knots 0 0 0 1 2 2 2
  spline S18 degree 2 poles (-2.9534, -190.2059) (-2.9534, -190.6876) (-2.4408, -191.2619) (-1.9592, -191.3915) knots 0 0 0 1 2 2 2
  spline S19 degree 2 poles (-1.9592, -191.3915) (-1.6381, -191.478) (-0.7057, -191.7003) (-0.3969, -191.7929) knots 0 0 0 1 2 2 2
  spline S20 degree 2 poles (-0.3969, -191.7929) (0.3873, -192.0337) (1.116, -193.0032) (1.116, -193.7134) knots 0 0 0 1 2 2 2
  spline S21 degree 2 poles (1.116, -193.7134) (1.116, -194.1641) (0.7516, -195.0286) (0.4244, -195.3312) knots 0 0 0 1 2 2 2
  spline S22 degree 2 poles (0.4244, -195.3312) (0.06, -195.6647) (-0.8662, -196.0228) (-1.564, -196.0228) knots 0 0 0 1 2 2 2
  line L38 (4.7222, -193.0156) -> (1.8385, -193.0156)
  line L39 (1.8385, -193.0156) -> (1.8385, -192.0893)
  line L40 (1.8385, -192.0893) -> (4.7222, -192.0893)
  line L41 (4.7222, -192.0893) -> (4.7222, -193.0156)
  line L42 (10.3662, -195.887) -> (5.951, -195.887)
  line L43 (5.951, -195.887) -> (5.951, -188.267)
  line L44 (5.951, -188.267) -> (6.9637, -188.267)
  line L45 (6.9637, -188.267) -> (6.9637, -194.9854)
  line L46 (6.9637, -194.9854) -> (10.3662, -194.9854)
  line L47 (10.3662, -194.9854) -> (10.3662, -195.887)
  spline S23 degree 2 poles (14.275, -195.2818) (14.1577, -195.3683) (13.7625, -195.677) (13.5772, -195.7696) knots 0 0 0 1 2 2 2
  spline S24 degree 2 poles (13.5772, -195.7696) (13.324, -195.9055) (12.8486, -196.0475) (12.4163, -196.0475) knots 0 0 0 1 2 2 2
  spline S25 degree 2 poles (12.4163, -196.0475) (12.0643, -196.0475) (11.4283, -195.782) (11.1875, -195.5412) knots 0 0 0 1 2 2 2
  spline S26 degree 2 poles (11.1875, -195.5412) (10.959, -195.3065) (10.6811, -194.6149) (10.6811, -194.2321) knots 0 0 0 1 2 2 2
  spline S27 degree 2 poles (10.6811, -194.2321) (10.6811, -193.6393) (11.1813, -192.7995) (11.7247, -192.5586) knots 0 0 0 1 2 2 2
  spline S28 degree 2 poles (11.7247, -192.5586) (12.2063, -192.3363) (13.5155, -192.1696) (14.275, -192.1264) knots 0 0 0 1 2 2 2
  line L48 (14.275, -192.1264) -> (14.275, -191.9411)
  spline S29 degree 2 poles (14.275, -191.9411) (14.275, -191.6077) (14.0712, -191.1939) (13.886, -191.0766) knots 0 0 0 1 2 2 2
  spline S30 degree 2 poles (13.886, -191.0766) (13.7007, -190.9593) (13.1697, -190.8852) (12.8856, -190.8852) knots 0 0 0 1 2 2 2
  spline S31 degree 2 poles (12.8856, -190.8852) (12.5522, -190.8852) (11.6506, -191.0828) (11.1998, -191.2742) knots 0 0 0 1 2 2 2
  line L49 (11.1998, -191.2742) -> (11.1442, -191.2742)
  line L50 (11.1442, -191.2742) -> (11.1442, -190.2924)
  spline S32 degree 2 poles (11.1442, -190.2924) (11.4098, -190.2183) (12.404, -190.033) (12.8918, -190.033) knots 0 0 0 1 2 2 2
  spline S33 degree 2 poles (12.8918, -190.033) (13.4846, -190.033) (14.2935, -190.2183) (14.6146, -190.4591) knots 0 0 0 1 2 2 2
  spline S34 degree 2 poles (14.6146, -190.4591) (14.9295, -190.6938) (15.2383, -191.4409) (15.2383, -191.9782) knots 0 0 0 1 2 2 2
  line L51 (15.2383, -191.9782) -> (15.2383, -195.887)
  line L52 (15.2383, -195.887) -> (14.275, -195.887)
  line L53 (14.275, -195.887) -> (14.275, -195.2818)
  line L54 (14.275, -194.4791) -> (14.275, -192.8921)
  spline S35 degree 2 poles (14.275, -192.8921) (13.9292, -192.923) (12.8856, -193.0279) (12.5583, -193.1267) knots 0 0 0 1 2 2 2
  spline S36 degree 2 poles (12.5583, -193.1267) (12.1755, -193.2441) (11.6753, -193.7319) (11.6753, -194.1641) knots 0 0 0 1 2 2 2
  spline S37 degree 2 poles (11.6753, -194.1641) (11.6753, -194.6581) (12.231, -195.1583) (12.7621, -195.1583) knots 0 0 0 1 2 2 2
  spline S38 degree 2 poles (12.7621, -195.1583) (13.2129, -195.1583) (13.9539, -194.7693) (14.275, -194.4791) knots 0 0 0 1 2 2 2
  spline S39 degree 2 poles (21.3825, -192.9353) (21.3825, -194.337) (20.024, -196.0475) (18.9989, -196.0475) knots 0 0 0 1 2 2 2
  spline S40 degree 2 poles (18.9989, -196.0475) (18.5358, -196.0475) (17.875, -195.819) (17.5539, -195.6214) knots 0 0 0 1 2 2 2
  line L55 (17.5539, -195.6214) -> (17.4922, -195.887)
  line L56 (17.4922, -195.887) -> (16.5906, -195.887)
  line L57 (16.5906, -195.887) -> (16.5906, -187.9273)
  line L58 (16.5906, -187.9273) -> (17.5539, -187.9273)
  line L59 (17.5539, -187.9273) -> (17.5539, -190.7679)
  spline S41 degree 2 poles (17.5539, -190.7679) (17.9183, -190.4406) (18.7642, -190.0083) (19.3015, -190.0083) knots 0 0 0 1 2 2 2
  spline S42 degree 2 poles (19.3015, -190.0083) (20.271, -190.0083) (21.3825, -191.5583) (21.3825, -192.9353) knots 0 0 0 1 2 2 2
  spline S43 degree 2 poles (20.3883, -193.0094) (20.3883, -191.9843) (19.7646, -190.9222) (19.073, -190.9222) knots 0 0 0 1 2 2 2
  spline S44 degree 2 poles (19.073, -190.9222) (18.684, -190.9222) (17.8812, -191.2927) (17.5539, -191.5768) knots 0 0 0 1 2 2 2
  line L60 (17.5539, -191.5768) -> (17.5539, -194.8557)
  spline S45 degree 2 poles (17.5539, -194.8557) (17.9183, -195.0348) (18.4802, -195.183) (18.8136, -195.183) knots 0 0 0 1 2 2 2
  spline S46 degree 2 poles (18.8136, -195.183) (19.5485, -195.183) (20.3883, -194.1394) (20.3883, -193.0094) knots 0 0 0 1 2 2 2
  point P0 (0, 0)
  constraints: 2 other
emboss "Emboss2" sketch "Sketch14" operation cut depth 2.54 direction (1, 0, 0)
sketch "Sketch15" plane through (0, -213.7841, 48.4212) normal (0, 0, 1) x (1, 0, 0)
  line L0 (20.32, 0) -> (20.32, 261.366) projected
  line L1 (16.002, 162.687) -> (20.32, 162.687)
  line L2 (20.32, 162.687) -> (20.32, 170.688)
  line L3 (20.32, 170.688) -> (16.002, 170.688)
  line L4 (16.002, 170.688) -> (16.002, 162.687)
  line L5 (20.32, 264.541) -> (0, 264.541) projected
  point P0 (0, 213.7841)
  point P1 (18.161, 170.688)
  dimension "d78" = 8.001
  dimension "d79" = 4.318
  dimension "d83" = 101.854
  constraints: 8 end point, 2 parallel, 1 horizontal, 1 midpoint, 1 perpendicular, 1 point on line
  measures "d78" distance of L3.end L1.start
  measures "d79" distance between parallel lines of L0 L4
  measures "d83" distance between parallel lines of L5 L1
extrude "Extrusion9" cut sketch "Sketch15" against normal blind 6.35